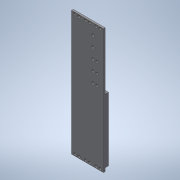
# Autodesk Inventor part: LeftBoxCover
Saved by Autodesk Inventor 2020 (Build 240168000, 168)
## iProperties
Created: 2019-06-03
Part Number: LeftBoxCover
Material: Generic
Document SubType Name: Modeling
Designer: LillaHunden
Density: 1 g/cm^3
Appearance: Default
Author: LillaHunden
Autodesk Inventor part; units mm, degrees
ref_plane "YZ Plane" through (0, 0, 0) normal (1, 0, 0) x (0, 1, 0)
ref_plane "XZ Plane" through (0, 0, 0) normal (0, 1, 0) x (-1, 0, 0)
ref_plane "XY Plane" through (0, 0, 0) normal (0, 0, 1) x (1, 0, 0)
sketch "Sketch1" plane through (0, 0, 0) normal (0, 0, 1) x (1, 0, 0)
  line L0 (67, 4) -> (76.9823, 4) construction
  line L1 (76.9823, 4) -> (76.9823, 12) construction
  line L2 (0, 12) -> (76.9823, 12) construction
  line L3 (0, 0) -> (0, 12) construction
  line L4 (67, 0) -> (0, 0) construction
  line L5 (67, 0) -> (67, 4) construction
  line L6 (67, -280) -> (67, -276) construction
  line L7 (67, -276) -> (0, -276) construction
  line L8 (0, -276) -> (0, -288) construction
  line L9 (76.9823, -288) -> (0, -288) construction
  line L10 (76.9823, -280) -> (76.9823, -288) construction
  line L11 (76.9823, -280) -> (67, -280) construction
  line L12 (76.9823, 12) -> (0, 12)
  line L13 (0, 12) -> (0, -288)
  line L14 (0, -288) -> (76.9823, -288)
  line L15 (76.9823, -288) -> (76.9823, 12)
  circle A0 centre (18, 7.95) radius 1.2295 projected
  circle A1 centre (43.4912, 7.95) radius 1.2295 projected
  circle A2 centre (68.9823, 7.95) radius 1.2295 projected
  circle A3 centre (58.9823, 7.95) radius 1.2295 projected
  circle A4 centre (33.4912, 7.95) radius 1.2295 projected
  circle A5 centre (8, 7.95) radius 1.2295 projected
  circle A6 centre (18, -283.95) radius 1.2295 projected
  circle A7 centre (43.4912, -283.95) radius 1.2295 projected
  circle A8 centre (68.9823, -283.95) radius 1.2295 projected
  circle A9 centre (33.4912, -283.95) radius 1.2295 projected
  circle A10 centre (8, -283.95) radius 1.2295 projected
  circle A11 centre (58.9823, -283.95) radius 1.2295 projected
  constraints: 8 end point, 2 parallel, 1 horizontal, 1 perpendicular
extrude "Extrusion1" add sketch "Sketch1" along normal blind 12 contours L15 L14 L13 L12 | A0 | A1 | A2 | A3 | A4 | A5 | A6 | A7 | A8 | A9 | A10 | A11
sketch "Sketch2" plane through (0, 0, 0) normal (0, 0, -1) x (-1, 0, 0)
  line L0 (-76.9823, -280) -> (-67, -280) construction
  line L1 (-67, -276) -> (0, -276) construction
  line L2 (-67, -280) -> (-67, -276) construction
  line L3 (0, -275.9) -> (-67.1, -275.9)
  line L4 (-67.1, -275.9) -> (-67.1, -279.9)
  line L5 (-67.1, -279.9) -> (-76.9823, -279.9)
  line L6 (0, 12) -> (0, -288) projected
  line L7 (-76.9823, 12) -> (0, 12) projected
  line L8 (-76.9823, -288) -> (-76.9823, 12) projected
  line L9 (0, -288) -> (-76.9823, -288) projected
  point P0 (0, 0)
  dimension "d2" = 0.1
  constraints: 6 end point, 2 other
  measures "d2" distance between parallel lines of L1 L3
extrude "Extrusion2" cut sketch "Sketch2" against normal blind 8 contours L6 L9 L8 L5 L4 L3
sketch "Sketch3" plane through (0, 0, 0) normal (0, 0, -1) x (-1, 0, 0)
  line L0 (-67, 4) -> (-76.9823, 4) construction
  line L1 (-67, 0) -> (0, 0) construction
  line L2 (-67, 0) -> (-67, 4) construction
  line L3 (-76.9823, 3.9) -> (-67.1, 3.9)
  line L4 (-67.1, 3.9) -> (-67.1, -0.1)
  line L5 (-67.1, -0.1) -> (0, -0.1)
  line L6 (-67.1, -275.9) -> (0, -275.9) projected
  line L7 (0, 12) -> (0, -275.9) projected
  line L8 (-76.9823, 12) -> (0, 12) projected
  line L9 (-76.9823, -279.9) -> (-76.9823, 12) projected
  line L10 (-76.9823, -279.9) -> (-67.1, -279.9) projected
  line L11 (-67.1, -279.9) -> (-67.1, -275.9) projected
  point P0 (0, -0.1)
  dimension "d5" = 0.1
  constraints: 6 end point, 2 other
  measures "d5" distance between parallel lines of L0 L3
extrude "Extrusion3" cut sketch "Sketch3" against normal up to surface (8 mm away) contours L9 L8 L7 L5 L4 L3
sketch "Sketch4" plane through (76.9823, -288, 12) normal (1, 0, 0) x (0, 0, -1)
  line L0 (4, 291.9) -> (4, 300) projected
  line L1 (12, 8.1) -> (12, 291.9) projected
  line L2 (4, 291.9) -> (12, 291.9)
  line L3 (12, 291.9) -> (12, 161.7)
  line L4 (12, 161.7) -> (4, 161.7)
  line L5 (4, 161.7) -> (4, 291.9)
  line L6 (197, 162) -> (4, 162) construction
  point P0 (12, 288)
  dimension "d8" = 0.3
  constraints: 8 end point, 2 parallel, 1 horizontal, 1 perpendicular, 1 point on line
  measures "d8" distance between parallel lines of L6 L4
ref_plane "Work Plane1" through (48, -120, -184.25) normal (-1, 0, 0) x (0, 0, 1)
extrude "Extrusion4" cut sketch "Sketch4" against normal up to surface (28.9823 mm away) draft 0.3
sketch "Sketch5" plane through (48, -126.4518, 8.1518) normal (1, 0, 0) x (0, 0, -1)
  arc A0 (6.828, 119.8758) -> (6.828, 114.6758) centre (6.828, 117.2758) ccw construction
  line L0 (6.828, 119.8758) -> (21.628, 119.8758) construction
  line L1 (21.628, 114.6758) -> (6.828, 114.6758) construction
  arc A1 (6.828, 72.7358) -> (6.828, 67.5358) centre (6.828, 70.1358) ccw construction
  line L2 (21.628, 67.5358) -> (6.828, 67.5358) construction
  line L3 (6.828, 72.7358) -> (21.628, 72.7358) construction
  line L4 (21.628, 111.6758) -> (6.828, 111.6758)
  arc A2 (6.828, 122.8758) -> (6.828, 111.6758) centre (6.828, 117.2758) ccw
  line L5 (6.828, 122.8758) -> (21.628, 122.8758)
  line L6 (21.628, 64.5358) -> (6.828, 64.5358)
  arc A3 (6.828, 75.7358) -> (6.828, 64.5358) centre (6.828, 70.1358) ccw
  line L7 (6.828, 75.7358) -> (21.628, 75.7358)
  line L8 (8.1518, 126.3518) -> (8.1518, 0) projected
  line L9 (8.1518, 111.6758) -> (8.1518, 122.8758)
  line L10 (8.1518, 75.7358) -> (8.1518, 64.5358)
  point P0 (8.1518, 126.4518)
  point P1 (8.1518, 64.5358)
  point P2 (8.1518, 75.7358)
  dimension "d11" = 3
  dimension "d12" = 3
  constraints: 12 end point, 8 point on line, 4 point on circle, 2 centre point, 4 other
  measures "d11" radial gap between concentric circles of A0 A2
  measures "d12" radial gap between concentric circles of A1 A3
extrude "Extrusion5" cut sketch "Sketch5" against normal blind 8.25
sketch "Sketch6" plane through (48, -126.4518, 8.1518) normal (1, 0, 0) x (0, 0, -1)
  line L0 (193.1518, 6.4518) -> (0.1518, 6.4518) construction
  line L1 (0.1518, 6.4518) -> (0.1518, 0.4518) construction
  line L2 (193.1518, 0.4518) -> (0.1518, 0.4518) construction
  line L3 (193.1518, 6.4518) -> (193.1518, 0.4518) construction
  line L4 (0.1518, 10.4518) -> (193.1518, 10.4518) construction
  line L5 (0.1518, 0.4518) -> (193.1518, 0.4518) construction
  line L6 (0.1518, 0.1518) -> (0, 0) projected
  line L7 (8.1518, 64.5358) -> (8.1518, 0) projected
  line L8 (0, 0) -> (8.1518, 0)
  line L9 (8.1518, 0) -> (8.1518, 10.7518)
  line L10 (8.1518, 10.7518) -> (0, 10.7518)
  line L11 (0, 10.7518) -> (0, 0)
  point P0 (8.1518, 126.4518)
  dimension "d15" = 0.3
  constraints: 8 end point, 2 parallel, 1 horizontal, 1 perpendicular, 1 point on line
  measures "d15" distance between parallel lines of L10 L4
extrude "Extrusion6" cut sketch "Sketch6" against normal through all
sketch "Sketch7" plane through (0, -275.9, 0) normal (0, -1, 0) x (1, 0, 0)
  point P0 (56.9823, 3)
  point P1 (46.9823, 3)
  point P2 (30, 3)
  point P3 (20, 3)
hole "Hole1" at (56.9823, -275.9, 3) at (46.9823, -275.9, 3) at (30, -275.9, 3) at (20, -275.9, 3) direction (0, 1, 0) diameter 2.459 depth 8 tip angle 120 thread size "M3x0.5" class "6H" standard "ISO Metric profile"
sketch "Sketch9" plane through (0, 0, 12) normal (0, 0, 1) x (1, 0, 0)
  line L0 (0, 12) -> (0, -288) projected
  line L1 (76.9823, -288) -> (76.9823, 12) projected
  line L2 (76.9823, -280) -> (76.9823, -288) construction
  line L3 (50.2323, -288) -> (43.7323, -288) construction
  line L4 (33.25, -288) -> (26.75, -288) construction
  line L5 (43.7323, -288) -> (33.25, -288) construction
  line L6 (0, -288) -> (76.9823, -288) construction
  point P0 (0, 0)
  point P1 (66.9823, -284)
  point P2 (10, -284)
  point P3 (38.4912, -284)
  point P4 (76.9823, -284)
  point P5 (38.4912, -288)
  dimension "d37" = 10
  dimension "d38" = 10
  constraints: 3 horizontal alignment, 2 end point, 2 midpoint, 1 collinear, 1 vertical alignment
  measures "d37" distance from line of L0 point (10, -284)
  measures "d38" distance from line of L1 point (66.982, -284)
sketch "Sketch13" plane through (0, 0, 12) normal (0, 0, 1) x (1, 0, 0)
  line L0 (76.9823, 3.9) -> (76.9823, 12) projected
  line L1 (0, 12) -> (0, -288) projected
  line L2 (33.4912, 7.95) -> (43.4912, 7.95) construction
  line L3 (76.9823, 12) -> (0, 12) projected
  line L4 (76.9823, -288) -> (76.9823, 12) projected
  line L5 (76.9823, -138) -> (0, -138) construction
  line L6 (76.9823, -279.9) -> (76.9823, -288)
  line L7 (33.4912, -283.95) -> (43.4912, -283.95) construction
  line L8 (76.9823, -288) -> (0, -288)
  point P0 (0, 0)
  point P1 (68.9823, 7.95)
  point P2 (58.9823, 7.95)
  point P3 (18, 7.95)
  point P4 (8, 7.95)
  point P5 (76.9823, 7.95)
  point P6 (38.4912, 7.95)
  point P7 (38.4912, 12)
  point P8 (0, -276)
  point P9 (68.9823, -283.95)
  point P10 (58.9823, -283.95)
  point P11 (18, -283.95)
  point P12 (8, -283.95)
  point P13 (76.9823, -283.95)
  point P14 (38.4912, -283.95)
  point P15 (38.4912, -288)
  dimension "d84" = 10
  dimension "d85" = 8
  dimension "d87" = 10
  dimension "d88" = 10
  dimension "d89" = 8
  constraints: 11 symmetric about line, 10 end point, 6 horizontal alignment, 5 midpoint, 1 horizontal, 1 vertical alignment
  measures "d84" distance of point (58.982, 7.95) point (68.982, 7.95)
  measures "d85" distance of point (76.982, 7.95) point (68.982, 7.95)
  measures "d87" distance of L2.start L2.end
  measures "d88" distance of point (8, 7.95) point (18, 7.95)
  measures "d89" distance from line of L1 point (8, 7.95)
sketch "Sketch14" plane through (0, 0, 12) normal (0, 0, 1) x (1, 0, 0)
  point P0 (68.9823, 7.95)
  point P1 (58.9823, 7.95)
  point P2 (43.4912, 7.95)
  point P3 (33.4912, 7.95)
  point P4 (18, 7.95)
  point P5 (8, 7.95)
hole "Hole6" at (68.9823, 7.95, 12) at (58.9823, 7.95, 12) at (43.4912, 7.95, 12) at (33.4912, 7.95, 12) at (18, 7.95, 12) at (8, 7.95, 12) direction (0, 0, -1) diameter 3.4 depth 4 countersink diameter 6.3 countersink angle 90
sketch "Sketch15" plane through (0, 0, 12) normal (0, 0, 1) x (1, 0, 0)
  point P0 (68.9823, -283.95)
  point P1 (68.9823, 7.95)
  point P2 (58.9823, 7.95)
  point P3 (43.4912, 7.95)
  point P4 (33.4912, 7.95)
  point P5 (18, 7.95)
  point P6 (8, 7.95)
  point P7 (33.4912, -283.95)
  point P8 (43.4912, -283.95)
  point P9 (8, -283.95)
  point P10 (18, -283.95)
  point P11 (58.9823, -283.95)
hole "Hole7" at (68.9823, -283.95, 12) at (68.9823, 7.95, 12) at (58.9823, 7.95, 12) at (43.4912, 7.95, 12) at (33.4912, 7.95, 12) at (18, 7.95, 12) at (8, 7.95, 12) at (33.4912, -283.95, 12) at (43.4912, -283.95, 12) at (8, -283.95, 12) at (18, -283.95, 12) at (58.9823, -283.95, 12) direction (0, 0, -1) diameter 3.4 depth 4 countersink diameter 6.3 countersink angle 90
sketch "Sketch16" plane through (0, 0, 12) normal (0, 0, 1) x (1, 0, 0)
  point P0 (61.5, -89.2459)
  point P1 (61.5, -64.2459)
  point P2 (61.5, -114.2459)
  point P3 (51.5, -114.2459)
  point P4 (51.5, -89.2459)
  point P5 (51.5, -64.2459)
  point P6 (51.5, -39.2459)
  point P7 (51.5, -14.2459)
hole "Hole9" at (61.5, -89.2459, 12) at (61.5, -64.2459, 12) at (61.5, -114.2459, 12) at (51.5, -114.2459, 12) at (51.5, -89.2459, 12) at (51.5, -64.2459, 12) at (51.5, -39.2459, 12) at (51.5, -14.2459, 12) direction (0, 0, -1) diameter 3.4 end up to surface countersink diameter 6.3 countersink angle 90
sketch "Sketch18" plane through (76.9823, 12, 8) normal (0, 0, -1) x (-1, 0, 0)
  circle A0 centre (26.1539, -10.7767) radius 4
  line L0 (28.9823, -7.9482) -> (14.8519, -22.0787) construction
  line L1 (28.9823, -12.1) -> (28.9823, -15.5759) projected
  point P0 (76.9823, -12)
  dimension "d113" = 8
  dimension "d114" = 45
  constraints: 2 end point, 1 coincident, 1 point on line, 3 other
  measures "d114" angle of L1 L0
extrude "Extrusion9" cut sketch "Sketch18" against normal up to surface surface through (76.9823, 3.9, 8) normal (0.005236, 0, 0.9999863)
sketch "Sketch19" plane through (0, 0, 0) normal (0, 0, -1) x (-1, 0, 0)
  arc A0 (-47.0537, -0.1) -> (-53.6863, 4.022) centre (-50.8284, 1.2233) ccw projected
  circle A1 centre (-50.8284, 1.2233) radius 4
  point P0 (0, 0)
  point P1 (-53.6863, 4.022)
  point P2 (-47.0537, -0.1)
  constraints: 1 centre point, 1 coincident
extrude "Extrusion10" cut sketch "Sketch19" against normal up to surface surface through (76.9823, 3.9, 8) normal (0.005236, 0, 0.9999863)
sketch "Sketch20" plane through (0, 0, 0) normal (0, 0, -1) x (-1, 0, 0)
  circle A0 centre (-50.8136, -123.6086) radius 4
  line L0 (-48, -115.7) -> (-48, -126.4518) construction
  line L1 (-48, -126.4518) -> (-76.9823, -126.3) construction
  line L2 (-48, -126.4518) -> (-53.6272, -120.7654) construction
  point P0 (0, 0)
  dimension "d119" = 8
  dimension "d120" = 45
  constraints: 2 end point, 1 coincident, 1 midpoint, 3 other
  measures "d120" angle of L1 L2
extrude "Extrusion11" cut sketch "Sketch20" against normal up to surface surface through (76.9823, 3.9, 8) normal (0.005236, 0, 0.9999863)
sketch "Sketch21" plane through (0, 0, 0) normal (0, 0, -1) x (-1, 0, 0)
  circle A0 centre (-64.2716, -278.7284) radius 4
  line L0 (-67.1, -279.9) -> (-67.1, -275.9) construction
  line L1 (-67.1, -275.9) -> (0, -275.9) construction
  line L2 (-67.1, -275.9) -> (-61.4431, -281.5569) construction
  point P0 (0, 0)
  dimension "d123" = 8
  dimension "d124" = 45
  constraints: 2 end point, 1 coincident, 1 midpoint, 3 other
  measures "d124" angle of L1 L2
extrude "Extrusion12" cut sketch "Sketch21" against normal up to surface (8 mm away)
equation "\"d11\" = d12"
body "Solid1"
